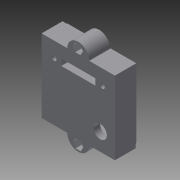
# Autodesk Inventor part: cameraPCBholder
Saved by Autodesk Inventor 2015 (Build 190159000, 159)
## iProperties
Created: 2015-03-20
Part Number: cameraPCBholder
Material: Generic
Document SubType Name: Modeling
Designer: Akovo_000
Density: 1 g/cm^3
Appearance: Default
Author: Akovo_000
Autodesk Inventor part; units mm, degrees
ref_plane "YZ Plane" through (0, 0, 0) normal (1, 0, 0) x (0, 1, 0)
ref_plane "XZ Plane" through (0, 0, 0) normal (0, 1, 0) x (-1, 0, 0)
ref_plane "XY Plane" through (0, 0, 0) normal (0, 0, 1) x (1, 0, 0)
sketch "Sketch1" plane through (0, 0, 0) normal (0, 1, 0) x (-1, 0, 0)
  line L0 (5.6174, 6.5261) -> (-19.9826, 6.5261)
  line L1 (-19.9826, 6.5261) -> (-19.9826, -19.0739)
  line L2 (-19.9826, -19.0739) -> (5.6174, -19.0739)
  line L3 (5.6174, -19.0739) -> (5.6174, 6.5261)
  line L4 (6.8174, 7.7261) -> (-21.1826, 7.7261)
  line L5 (-21.1826, 7.7261) -> (-21.1826, -20.2739)
  line L6 (-21.1826, -20.2739) -> (6.8174, -20.2739)
  line L7 (6.8174, -20.2739) -> (6.8174, 7.7261)
  circle A0 centre (4.0674, 4.9761) radius 0.95
  circle A1 centre (-18.4326, 4.9761) radius 0.95
  circle A2 centre (-18.4326, -17.5239) radius 0.95
  circle A3 centre (4.0674, -17.5239) radius 0.95
  arc A4 (-11.3826, -20.2739) -> (-2.9826, -20.2739) centre (-7.1826, -20.2739) ccw
  arc A5 (-2.9826, 7.7261) -> (-11.3826, 7.7261) centre (-7.1826, 7.7261) ccw
  line L8 (-11.3826, -20.2739) -> (-2.9826, -20.2739)
  line L9 (-2.9826, 7.7261) -> (-11.3826, 7.7261)
  point P0 (0, 0)
  dimension "d0" = 25.6
  dimension "d1" = 25.6
  dimension "d2" = 28
  dimension "d3" = 28
  dimension "d4" = 1.2
  dimension "d5" = 1.2
  dimension "d6" = 1.2
  dimension "d7" = 1.2
  dimension "d8" = 25.6
  dimension "d9" = 25.6
  dimension "d10" = 1.9
  dimension "d11" = 1.55
  dimension "d12" = 1.55
  dimension "d13" = 1.9
  dimension "d14" = 1.55
  dimension "d15" = 1.55
  dimension "d16" = 1.9
  dimension "d17" = 1.55
  dimension "d18" = 1.55
  dimension "d19" = 1.9
  dimension "d20" = 1.55
  dimension "d21" = 1.55
  dimension "d22" = 22.5
  dimension "d23" = 22.5
  dimension "d160" = 4.2
  dimension "d161" = 4.2
  constraints: 20 end point, 6 centre point, 4 parallel, 4 point on circle, 2 collinear, 2 horizontal, 2 midpoint, 2 perpendicular, 2 point on line
  measures "d0" distance of L2.end L1.end
  measures "d1" distance of L1.end L0.end
  measures "d2" distance of L6.end L5.end
  measures "d3" distance of L5.end L4.end
  measures "d4" distance between parallel lines of L3 L7
  measures "d5" distance between parallel lines of L4 L0
  measures "d6" distance between parallel lines of L6 L2
  measures "d7" distance between parallel lines of L5 L1
  measures "d8" distance between parallel lines of L2 L0
  measures "d9" distance between parallel lines of L1 L3
  measures "d10" diameter of A0
  measures "d11" distance from line of L3 A0.centre
  measures "d12" distance from line of L0 A0.centre
  measures "d13" diameter of A1
  measures "d14" distance from line of L0 A1.centre
  measures "d15" distance from line of A1.centre L1
  measures "d16" diameter of A2
  measures "d17" distance from line of A2.centre L1
  measures "d18" distance from line of L2 A2.centre
  measures "d19" diameter of A3
  measures "d20" distance from line of L3 A3.centre
  measures "d21" distance from line of L2 A3.centre
  measures "d22" distance of A3.centre A0.centre
  measures "d23" distance of A1.centre A0.centre
  measures "d160" radius of A4
  measures "d161" radius of A5
extrude "PCB container" add sketch "Sketch1" along normal blind 5.5 contours L7 L6 L5 L4 | L4 A5 | A4 L6
sketch "Sketch2" plane through (0, 0, 0) normal (0, -1, 0) x (1, 0, 0)
  line L0 (21.1826, -20.2739) -> (-6.8174, -20.2739)
  line L1 (-6.8174, -20.2739) -> (-6.8174, 7.7261)
  line L2 (-6.8174, 7.7261) -> (21.1826, 7.7261)
  line L3 (21.1826, 7.7261) -> (21.1826, -20.2739)
  line L4 (19.9826, -19.0739) -> (-5.6174, -19.0739)
  line L5 (-5.6174, -19.0739) -> (-5.6174, 6.5261)
  line L6 (-5.6174, 6.5261) -> (19.9826, 6.5261)
  line L7 (19.9826, 6.5261) -> (19.9826, -19.0739)
  circle A0 centre (15.5826, -13.5739) radius 2.55
  circle A1 centre (16.4076, 1.9311) radius 0.925
  circle A2 centre (-2.0424, 1.9311) radius 0.925
  line L8 (13.6826, 0.7061) -> (0.6826, 0.7061)
  line L9 (0.6826, 0.7061) -> (0.6826, 3.1561)
  line L10 (0.6826, 3.1561) -> (13.6826, 3.1561)
  line L11 (13.6826, 3.1561) -> (13.6826, 0.7061)
  line L12 (9.0818, -22.1627) -> (8.1068, -23.8514)
  line L13 (8.1068, -23.8514) -> (6.1568, -23.8514)
  line L14 (6.1568, -23.8514) -> (5.1818, -22.1627)
  line L15 (5.1818, -22.1627) -> (6.1568, -20.4739)
  line L16 (6.1568, -20.4739) -> (8.1068, -20.4739)
  line L17 (8.1068, -20.4739) -> (9.0818, -22.1627)
  line L18 (8.9714, 9.6148) -> (7.9964, 7.9261)
  line L19 (7.9964, 7.9261) -> (6.0464, 7.9261)
  line L20 (6.0464, 7.9261) -> (5.0714, 9.6148)
  line L21 (5.0714, 9.6148) -> (6.0464, 11.3036)
  line L22 (6.0464, 11.3036) -> (7.9964, 11.3036)
  line L23 (7.9964, 11.3036) -> (8.9714, 9.6148)
  arc A3 (2.9826, -20.2739) -> (11.3826, -20.2739) centre (7.1826, -20.2739) ccw
  arc A4 (11.3826, 7.7261) -> (2.9826, 7.7261) centre (7.1826, 7.7261) ccw
  line L24 (2.9826, -20.2739) -> (11.3826, -20.2739)
  line L25 (2.9826, 7.7261) -> (11.3826, 7.7261)
  point P0 (0, 0)
  point P1 (0, 0)
  point P2 (7.1318, -22.1627)
  point P3 (7.0214, 9.6148)
  dimension "d26" = 5.1
  dimension "d27" = 5.5
  dimension "d28" = 4.4
  dimension "d29" = 1.85
  dimension "d30" = 1.85
  dimension "d35" = 2.725
  dimension "d36" = 2.725
  dimension "d37" = 13
  dimension "d38" = 2.45
  dimension "d39" = 1.225
  dimension "d40" = 1.225
  dimension "d41" = 18.45
  dimension "d42" = 19.3
  dimension "d43" = 1.2
  dimension "d44" = 1.2
  dimension "d45" = 19.3
  dimension "d46" = 3.37
  dimension "d47" = 1.2
  dimension "d48" = 1.2
  dimension "d49" = 19.78
  dimension "d50" = 25.6
  dimension "d164" = 1.95
  dimension "d165" = 1.95
  dimension "d166" = 0.2
  dimension "d167" = 0.2
  dimension "d168" = 4.2
  dimension "d169" = 0.6225
  dimension "d170" = 0.6225
  constraints: 52 end point, 6 parallel, 5 centre point, 5 horizontal, 4 point on circle, 3 perpendicular, 2 midpoint, 1 point on line, 26 other
  measures "d26" diameter of A0
  measures "d27" distance from line of L4 A0.centre
  measures "d28" distance from line of L7 A0.centre
  measures "d29" diameter of A1
  measures "d30" diameter of A2
  measures "d35" distance from line of A1.centre L11
  measures "d36" distance from line of A2.centre L9
  measures "d37" distance between parallel lines of L9 L11
  measures "d38" distance between parallel lines of L10 L8
  measures "d39" distance from line of A1.centre L10
  measures "d40" distance from line of L10 A2.centre
  measures "d41" distance of A2.centre A1.centre
  measures "d42" distance between parallel lines of L5 L11
  measures "d43" distance between parallel lines of L1 L5
  measures "d44" distance between parallel lines of L3 L7
  measures "d45" distance between parallel lines of L7 L9
  measures "d46" distance between parallel lines of L6 L10
  measures "d47" distance between parallel lines of L4 L0
  measures "d48" distance between parallel lines of L2 L6
  measures "d49" distance between parallel lines of L4 L8
  measures "d50" distance between parallel lines of L6 L4
  measures "d164" distance of L12.start point (7.132, -22.163)
  measures "d165" distance of L18.start point (7.021, 9.615)
  measures "d166" distance between parallel lines of L0 L16
  measures "d167" distance between parallel lines of L2 L19
  measures "d168" radius of A3
  measures "d169" distance edge to line of A3 L13
  measures "d170" distance edge to line of A4 L22
extrude "BackSide" add sketch "Sketch2" along normal blind 2.5 contours L0 L1 L2 L3 | A3 L0 | L2 A4 | L4 L5 L6 L7
sketch "BoardSupport" plane through (0, 0, 0) normal (0, 1, 0) x (1, 0, 0)
  line L0 (-2.6174, 17.5739) -> (-2.6174, 19.0739)
  line L1 (-4.1174, 16.0739) -> (-5.6174, 16.0739)
  arc A0 (-4.1174, 16.0739) -> (-2.6174, 17.5739) centre (-4.1174, 17.5739) ccw
  line L2 (18.5051, 16.0741) -> (19.9826, 16.0741)
  arc A1 (16.9826, 17.5739) -> (18.5051, 16.0741) centre (18.4826, 17.5739) ccw
  line L3 (16.9826, 17.5739) -> (16.9826, 19.0739)
  line L4 (-4.1174, -3.5261) -> (-5.6174, -3.5261)
  arc A2 (-2.6174, -5.0261) -> (-4.1174, -3.5261) centre (-4.1174, -5.0261) ccw
  line L5 (16.9826, -5.0261) -> (16.9826, -6.5261)
  arc A3 (18.4826, -3.5261) -> (16.9826, -5.0261) centre (18.4826, -5.0261) ccw
  line L6 (18.4826, -3.5261) -> (19.9826, -3.5261)
  line L7 (-2.6174, -5.0261) -> (-2.6174, -6.5261)
  line L8 (-5.6174, -3.5261) -> (-5.6174, -6.5261)
  line L9 (-5.6174, 16.0739) -> (-5.6174, 19.0739)
  line L10 (-5.6174, 19.0739) -> (-2.6174, 19.0739)
  line L11 (16.9826, 19.0739) -> (19.9826, 19.0739)
  line L12 (19.9826, 19.0739) -> (19.9826, 16.0741)
  line L13 (16.9826, -6.5261) -> (19.9826, -6.5261)
  line L14 (19.9826, -6.5261) -> (19.9826, -3.5261)
  line L15 (-5.6174, -6.5261) -> (-2.6174, -6.5261)
  circle A4 centre (-4.1174, 17.5739) radius 0.925
  circle A5 centre (18.4826, 17.5739) radius 0.925
  circle A6 centre (-4.1174, -5.0261) radius 0.925
  circle A7 centre (18.4826, -5.0261) radius 0.925
  point P0 (0, 0)
  point P1 (0, 0)
  dimension "d61" = 1.5
  dimension "d62" = 25.6
  dimension "d63" = 25.6
  dimension "d64" = 25.6
  dimension "d65" = 25.6
  dimension "d67" = 1.5
  dimension "d68" = 1.5
  dimension "d69" = 1.5
  dimension "d93" = 1.85
  dimension "d94" = 1.85
  dimension "d95" = 1.85
  dimension "d96" = 1.85
  dimension "d101" = 1.5
  dimension "d102" = 1.5
  dimension "d103" = 1.5
  dimension "d104" = 1.5
  dimension "d105" = 1.5
  dimension "d106" = 1.5
  dimension "d107" = 1.5
  dimension "d108" = 1.5
  dimension "d109" = 1.5
  dimension "d110" = 1.5
  dimension "d111" = 1.5
  constraints: 32 end point, 8 centre point, 8 point on circle, 4 coincident, 2 perpendicular, 1 horizontal
  measures "d61" distance of L0.start A0.centre
  measures "d62" distance between parallel lines of L12 L9
  measures "d63" distance between parallel lines of L15 L10
  measures "d64" distance between parallel lines of L13 L11
  measures "d65" distance between parallel lines of L8 L14
  measures "d67" distance of L4.start A2.centre
  measures "d68" distance of L6.start A3.centre
  measures "d69" distance of L2.start A1.centre
  measures "d93" diameter of A4
  measures "d94" diameter of A5
  measures "d95" diameter of A6
  measures "d96" diameter of A7
  measures "d101" distance from line of L11 A1.centre
  measures "d102" distance from line of A0.centre L10
  measures "d103" distance from line of L9 A0.centre
  measures "d104" distance from line of L12 A1.centre
  measures "d105" distance from line of L13 A3.centre
  measures "d106" distance from line of L14 A3.centre
  measures "d107" distance from line of L15 A2.centre
  measures "d108" distance from line of A2.centre L8
  measures "d109" distance from line of L1 A0.centre
  measures "d110" distance from line of A1.centre L3
  measures "d111" distance of L5.start A3.centre
extrude "pcbSUPPORT" add sketch "BoardSupport" along normal blind 2
hole "PCBHole1" at (-4.1174, 0, -17.5739) direction (0, -1, 0) diameter 1.85 depth 2
hole "PCBhole2" at (18.4826, 0, 5.0261) direction (0, -1, 0) diameter 1.85 depth 2
hole "PCBHole3" at (-4.1174, 0, 5.0261) direction (0, -1, 0) diameter 1.85 depth 2
hole "PCBhole4" at (18.4826, 0, -17.5739) direction (0, -1, 0) diameter 1.85 depth 2
sketch "Sketch7" plane through (0, 5.5, 0) normal (0, 1, 0) x (1, 0, 0)
  line L0 (19.9826, -6.5261) -> (-5.6174, -6.5261)
  line L1 (-5.6174, -6.5261) -> (-5.6174, 19.0739)
  line L2 (-5.6174, 19.0739) -> (19.9826, 19.0739)
  line L3 (19.9826, 19.0739) -> (19.9826, -6.5261)
  line L4 (-6.0174, 19.4739) -> (20.3826, 19.4739)
  line L5 (20.3826, 19.4739) -> (20.3826, -6.9261)
  line L6 (20.3826, -6.9261) -> (-6.0174, -6.9261)
  line L7 (-6.0174, -6.9261) -> (-6.0174, 19.4739)
  point P0 (0, 0)
  dimension "d150" = 26.4
  dimension "d151" = 26.4
  dimension "d152" = 0.4
  dimension "d153" = 25.6
  dimension "d154" = 25.6
  dimension "d155" = 0.4
  dimension "d156" = 0.4
  dimension "d157" = 0.4
  constraints: 16 end point, 4 parallel, 2 horizontal, 2 perpendicular
  measures "d150" distance of L5.end L6.end
  measures "d151" distance of L4.end L5.end
  measures "d152" distance between parallel lines of L7 L1
  measures "d153" distance between parallel lines of L1 L3
  measures "d154" distance between parallel lines of L0 L2
  measures "d155" distance between parallel lines of L3 L5
  measures "d156" distance between parallel lines of L6 L0
  measures "d157" distance between parallel lines of L4 L2
extrude "Director" add sketch "Sketch7" along normal blind 1
sketch "Sketch9" plane through (0, -2.5, 0) normal (0, -1, 0) x (1, 0, 0)
  circle A0 centre (7.0214, 9.6148) radius 0.925
  circle A1 centre (7.1318, -22.1627) radius 0.925
  line L0 (9.0818, -22.1627) -> (8.1068, -23.8514)
  line L1 (6.1568, -23.8514) -> (5.1818, -22.1627)
  line L2 (5.1818, -22.1627) -> (6.1568, -20.4739)
  line L3 (6.1568, -20.4739) -> (8.1068, -20.4739)
  line L4 (8.1068, -20.4739) -> (9.0818, -22.1627)
  line L5 (8.9714, 9.6148) -> (7.9964, 7.9261)
  line L6 (7.9964, 7.9261) -> (6.0464, 7.9261)
  line L7 (6.0464, 7.9261) -> (5.0714, 9.6148)
  line L8 (5.0714, 9.6148) -> (6.0464, 11.3036)
  line L9 (6.0464, 11.3036) -> (7.9964, 11.3036)
  line L10 (7.9964, 11.3036) -> (8.9714, 9.6148)
  arc A2 (11.3826, 7.7261) -> (2.9826, 7.7261) centre (7.1826, 7.7384) ccw
  arc A3 (2.9826, -20.2739) -> (11.3826, -20.2739) centre (7.1826, -20.2739) ccw
  line L11 (11.3826, 7.7261) -> (2.9826, 7.7261)
  line L12 (2.9826, -20.2739) -> (11.3826, -20.2739)
  line L13 (20.3826, -19.4739) -> (-6.0174, -19.4739) projected
  line L14 (3.4251, 9.6148) -> (10.9402, 9.6148)
  point P0 (0, 0)
  dimension "d171" = 1.85
  dimension "d172" = 1.85
  dimension "d173" = 1.6887
  dimension "d174" = 1.6887
  dimension "d175" = 1.6887
  dimension "d186" = 1.8887
  dimension "d188" = 3.9188
  dimension "d189" = 3.5962
  dimension "d190" = 1.8887
  dimension "d191" = 3.9
  dimension "d192" = 1.8887
  dimension "d193" = 4.2
  dimension "d194" = 7.5151
  constraints: 28 end point, 6 point on circle, 4 centre point, 2 horizontal, 1 parallel
  measures "d171" diameter of A0
  measures "d172" diameter of A1
  measures "d173" distance from line of L0 A1.centre
  measures "d174" distance from line of L3 A1.centre
  measures "d175" distance from line of A1.centre L1
  measures "d186" distance from line of L12 A1.centre
  measures "d188" distance of A0.centre L14.end
  measures "d189" distance of A0.centre L14.start
  measures "d190" distance between parallel lines of L11 L14
  measures "d191" distance of L7.end L5.start
  measures "d192" distance from line of L11 A0.centre
  measures "d193" radius of A2
  measures "d194" distance of L14.start L14.end
hole "Hole5" at (7.0214, -2.5, 9.6148) at (7.1318, -2.5, -22.1627) direction (0, 1, 0) diameter 1.85 end through all
body "Solid1"
